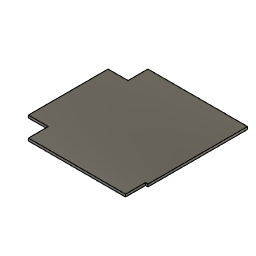
_Shelf1_2Edge.f91778a1-98cf-41b9-a237-7004ff5904d3 (Autodesk Fusion 360 design; units mm, degrees)
Autodesk Fusion 360 part; units mm, degrees
note: some values were not read from the file. Set by a fixed rule: which sketch regions a step uses.
sketch "Sketch1" plane through (0, 0, 0) normal (0, 0, 1) x (1, 0, 0)
  line L0 (0, 0) -> (0, 304.8)
  line L1 (0, 304.8) -> (304.8, 304.8)
  line L2 (304.8, 304.8) -> (304.8, 0)
  line L3 (304.8, 0) -> (0, 0)
  line L4 (0, 0) -> (50.8, 0)
  line L5 (50.8, 0) -> (50.8, 50.8)
  line L6 (50.8, 50.8) -> (0, 50.8)
  line L7 (0, 50.8) -> (0, 0)
  line L8 (0, 304.8) -> (50.8, 304.8)
  line L9 (50.8, 304.8) -> (50.8, 254)
  line L10 (50.8, 254) -> (0, 254)
  line L11 (0, 254) -> (0, 304.8)
  line L12 (304.8, 0) -> (298.45, 0)
  line L13 (298.45, 0) -> (298.45, 50.8)
  line L14 (298.45, 50.8) -> (304.8, 50.8)
  line L15 (304.8, 50.8) -> (304.8, 0)
  dimension "d2" = 304.8
  dimension "d3" = 304.8
  dimension "d10" = 50.8
  dimension "d13" = 50.8
  dimension "d14" = 6.35
  dimension "d17" = 50.8
  constraint coincident L0.start L3.end
  constraint vertical L0
  constraint perpendicular L0 L1
  constraint perpendicular L1 L2
  constraint perpendicular L0 L3
  constraint horizontal L4
  constraint vertical L5
  constraint horizontal L6
  constraint vertical L7
  constraint horizontal L8
  constraint vertical L9
  constraint horizontal L10
  constraint vertical L11
  constraint collinear L5 L9
  constraint horizontal L12
  constraint vertical L13
  constraint horizontal L14
  constraint vertical L15
  constraint collinear L6 L14
  measures "d2" distance of L0.start L0.end
  measures "d3" distance of L0.end L1.end
  measures "d10" distance of L0.start L4.end
  measures "d13" distance of L4.end L5.end
  measures "d14" distance of L13.end L14.end
  measures "d17" distance of L0.end L10.end
extrude "Extrude1" add sketch "Sketch1" along normal blind 6.35 contours L0 L1 L2 L3 L5 L6 L9 L10 L13 L14
